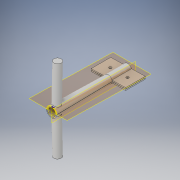
# Autodesk Inventor part: golfhandle
Saved by Autodesk Inventor 2018 (Build 220112000, 112)
## iProperties
Created: 2019-04-25
Part Number: golfhandle
Material: Generic
Document SubType Name: Modeling
Designer: F8PLTW
Density: 1 g/cm^3
Appearance: Default
Author: F8PLTW
Autodesk Inventor part; units mm, degrees
ref_plane "YZ Plane" through (0, 0, 0) normal (1, 0, 0) x (0, 1, 0)
ref_plane "XZ Plane" through (0, 0, 0) normal (0, 1, 0) x (-1, 0, 0)
ref_plane "XY Plane" through (0, 0, 0) normal (0, 0, 1) x (1, 0, 0)
sketch "Sketch1" plane through (0, 0, 0) normal (0, 0, 1) x (1, 0, 0)
  circle A0 centre (-3.872676, 4.498262) radius 10.795
  point P0 (0, 0)
  dimension "d0" = 21.59
  constraints: 1 centre point
  measures "d0" diameter of A0
extrude "Extrusion1" add sketch "Sketch1" along normal blind 2.54
ref_plane "Work Plane1" through (-3.872676, 4.498262, 156.718) normal (0, 0, 1) x (1, 0, 0)
sketch "Sketch2" plane through (-3.872676, 4.498262, 156.718) normal (0, 0, 1) x (1, 0, 0)
  circle A0 centre (0, 0) radius 13.716
  point P0 (3.872676, -4.498262)
  dimension "d4" = 27.432
  constraints: 1 centre point
  measures "d4" diameter of A0
loft "Loft1" add profiles "Sketch2" section 1 edges at (-14.667676, 4.498262, 2.54)
sketch "Sketch3" plane through (-3.872676, 4.498262, 0) normal (0, 0, -1) x (-1, 0, 0)
  circle A0 centre (0, 0) radius 10.795
  point P0 (-3.872676, -4.498262)
  dimension "d11" = 21.59
  constraints: 1 centre point
  measures "d11" diameter of A0
extrude "Extrusion2" add sketch "Sketch3" along normal blind 50.8
sketch "Sketch4" plane through (-3.872676, 4.498262, -50.8) normal (0, 0, -1) x (-1, 0, 0)
  point P0 (-3.872676, -4.498262)
sketch "Sketch5" plane through (-3.872676, 4.498262, -50.8) normal (0, 0, -1) x (-1, 0, 0)
  circle A0 centre (0, 0) radius 7.874
  point P0 (-3.872676, -4.498262)
  dimension "d12" = 15.748
  constraints: 1 centre point
  measures "d12" diameter of A0
extrude "Extrusion3" cut sketch "Sketch5" against normal blind 50.8
sketch "Sketch6" plane through (-3.872676, 4.498262, 0) normal (0, 0, -1) x (-1, 0, 0)
  circle A0 centre (0, 0) radius 7.62
  point P0 (-3.872676, -4.498262)
  constraints: 1 centre point
sketch "Sketch7" plane through (-3.872676, 4.498262, 156.718) normal (0, 0, 1) x (1, 0, 0)
  circle A0 centre (0, 0) radius 11.176
  point P0 (3.872676, -4.498262)
  dimension "d15" = 22.352
  constraints: 1 centre point
  measures "d15" diameter of A0
loft "Loft2" cut profiles "Sketch6", "Sketch7"
sketch "Sketch8" plane through (-3.872676, 4.498262, 0) normal (0, 0, -1) x (-1, 0, 0)
  circle A0 centre (0, 0) radius 7.874
  point P0 (-3.872676, -4.498262)
  constraints: 1 centre point
extrude "Extrusion4" cut sketch "Sketch8" against normal blind 2.54
sketch "Sketch9" plane through (-3.872676, 4.498262, 156.718) normal (0, 0, 1) x (1, 0, 0)
  line L0 (-5.096602, 0.25034) -> (248.903398, 0.25034)
  line L1 (248.903398, 0.25034) -> (248.903398, -0.25766)
  line L2 (248.903398, -0.25766) -> (-5.096602, -0.25766)
  line L3 (-5.096602, 0.25034) -> (-18.65647, 0.25034)
  line L4 (-5.096602, -0.25766) -> (-18.65647, -0.25766)
  line L5 (-18.65647, -0.25766) -> (-18.65647, 0.25034)
  point P0 (3.872676, -4.498262)
  dimension "d24" = 0.508
  dimension "d25" = 254
  constraints: 12 end point, 3 horizontal, 2 perpendicular, 1 parallel
  measures "d24" distance between parallel lines of L2 L0
  measures "d25" distance of L0.start L0.end
extrude "Extrusion5" cut sketch "Sketch9" against normal blind 228.6
ref_plane "Work Plane2" through (6.919421, 4.748602, 0) normal (0.9997311, 0.0231904, 0) x (-0.0231904, 0.9997311, 0)
sketch "Sketch10" plane through (6.919421, 4.748602, 0) normal (0.9997311, 0.0231904, 0) x (-0.0231904, 0.9997311, 0)
  line L0 (10.795, 2.54) -> (0, 2.54)
  line L1 (-0.075087, -50.8) -> (-7.874, -50.8)
  line L2 (3.133931, 2.54) -> (-0.075087, 2.54)
  line L3 (-0.075087, 2.54) -> (-0.075087, -50.8)
  line L4 (-0.075087, -50.8) -> (3.133931, -50.8)
  line L5 (3.133931, -50.8) -> (3.133931, 2.54)
  line L6 (-0.435537, 2.54) -> (-3.635937, 2.54)
  line L7 (-3.635937, 2.54) -> (-3.635937, -50.8)
  line L8 (-3.635937, -50.8) -> (-0.435537, -50.8)
  line L9 (-0.435537, -50.8) -> (-0.435537, 2.54)
  point P0 (-4.586861, 0)
  point P1 (0.500546, 2.54)
  point P2 (-0.440094, -50.8)
  dimension "d26" = 3.2004
  constraints: 16 end point, 4 parallel, 2 horizontal, 2 perpendicular, 2 point on line
  measures "d26" distance of L8.end L7.end
extrude "Extrusion6" add sketch "Sketch10" along normal mid plane 114.3
sketch "Sketch11" plane through (-50.287887, 6.556359, 2.54) normal (-0.0231904, 0.9997311, 0) x (0.9997311, 0.0231904, 0)
  circle A0 centre (24.391895, 27.825278) radius 3.429
  point P0 (50.122318, 2.54)
  dimension "d29" = 6.858
  constraints: 1 centre point
  measures "d29" diameter of A0
extrude "Extrusion7" cut sketch "Sketch11" against normal blind 50.8
sketch "Sketch12" plane through (6.381947, 7.870908, 2.54) normal (-0.0231904, 0.9997311, 0) x (0.9997311, 0.0231904, 0)
  line L0 (-18.20372, 0) -> (57.614922, 0)
  line L1 (-18.20372, 53.34) -> (57.614922, 53.34)
  line L2 (57.614922, 0) -> (37.396963, 0)
  line L3 (37.396963, 0) -> (37.396963, 53.34)
  line L4 (37.396963, 53.34) -> (57.614922, 53.34)
  line L5 (57.614922, 53.34) -> (57.614922, 0)
  point P0 (-6.56276, 2.54)
  constraints: 8 end point, 2 parallel, 1 horizontal, 1 perpendicular, 1 point on line
extrude "Extrusion8" cut sketch "Sketch12" against normal blind 50.8
sketch "Sketch13" plane through (6.381947, 7.870908, 2.54) normal (-0.0231904, 0.9997311, 0) x (0.9997311, 0.0231904, 0)
  circle A0 centre (15.500044, 27.091091) radius 3.429
  point P0 (-6.56276, 2.54)
  dimension "d34" = 6.858
  constraints: 1 centre point
  measures "d34" diameter of A0
extrude "Extrusion9" cut sketch "Sketch13" against normal blind 50.8
sketch "Sketch14" plane through (-3.872676, 4.498262, -50.8) normal (0, 0, -1) x (-1, 0, 0)
  circle A0 centre (0, 0) radius 7.874
  point P0 (-3.872676, -4.498262)
  constraints: 1 centre point
extrude "Extrusion10" cut sketch "Sketch14" against normal blind 63.5
sketch "Sketch15" plane through (-3.872676, 4.498262, -50.8) normal (0, 0, -1) x (-1, 0, 0)
  arc A0 (10.790094, -0.325401) -> (10.791925, -0.25766) centre (0, 0) ccw
  line L0 (-7.873266, 0.107526) -> (-47.715946, 1.031742)
  line L1 (10.791925, -0.25766) -> (-7.873266, 0.107526)
  arc A1 (-7.869783, -0.25766) -> (7.869783, -0.25766) centre (0, 0) ccw
  arc A2 (10.773209, -0.685557) -> (10.790094, -0.325401) centre (0, 0) ccw
  line L2 (-7.869783, -0.25766) -> (10.773209, -0.685557)
  line L3 (10.773209, -0.685557) -> (10.790094, -0.325401)
  line L4 (-7.873266, 0.107526) -> (-7.869783, -0.25766)
  point P0 (-3.872676, -4.498262)
  constraints: 8 end point
sketch "Sketch15 outline for Extrusion11" plane through (-3.872676, 4.498262, -50.8) normal (0, 0, -1) x (-1, 0, 0)
  arc A0 (10.790094, -0.325401) -> (10.791925, -0.25766) centre (0, 0) ccw
  line L0 (10.773209, -0.685557) -> (10.790094, -0.325401)
  line L1 (-7.869783, -0.25766) -> (10.773209, -0.685557)
  line L2 (-7.873266, 0.107526) -> (-7.869783, -0.25766)
  line L3 (10.791925, -0.25766) -> (-7.873266, 0.107526)
extrude "Extrusion11" cut sketch "Sketch15 outline for Extrusion11" against normal blind 304.8
sketch "Sketch16" plane through (-3.872676, 4.498262, 156.718) normal (0, 0, 1) x (1, 0, 0)
  arc A0 (13.713715, 0.25034) -> (-13.713715, 0.25034) centre (0, 0) ccw
  line L0 (0, 13.716) -> (8.803339, 13.716)
  point P0 (3.872676, -4.498262)
  constraints: 2 end point, 1 horizontal, 1 point on circle, 1 tangent
sketch "Sketch17" plane through (-3.872676, 4.498262, 156.718) normal (0, 0, 1) x (1, 0, 0)
  arc A0 (11.173196, 0.25034) -> (-11.173196, 0.25034) centre (0, 0) ccw
  line L0 (0, 11.176) -> (3.327889, 11.176)
  point P0 (3.872676, -4.498262)
  constraints: 2 end point, 1 horizontal, 1 point on circle, 1 tangent
ref_plane "Work Plane4" through (-3.872676, 15.674262, 156.718) normal (0, 0.9997427, -0.0226846) x (-1, 0, 0)
sketch "Sketch18" plane through (-3.872676, 15.674262, 156.718) normal (0, 0.9997427, -0.0226846) x (-1, 0, 0)
  ellipse E0 centre (0, -0.253523) end of major axis (13.716, -0.253523) minor radius 0.311142 (-13.71358, -0.259368) -> (13.71358, -0.259368) ccw
  line L0 (0, -0.253523) -> (0, -214.964518) construction
  circle A0 centre (0, -13.939044) radius 10.16
  point P0 (-3.872676, -157.033236)
  dimension "d41" = 20.32
  constraints: 2 end point, 1 centre point, 1 point on line, 1 vertical, 1 other
  measures "d41" diameter of A0
extrude "Extrusion12" add sketch "Sketch18" along normal blind 101.6
mirror "Mirror1" about plane through (-8.969278, 4.748602, 156.718) normal (0, -1, 0) of "Extrusion12"
sketch "Sketch19" plane through (-3.872676, 4.498262, 156.718) normal (0, 0, 1) x (1, 0, 0)
  circle A0 centre (0, 0) radius 11.176
  point P0 (3.872676, -4.498262)
  constraints: 1 centre point
extrude "Extrusion13" cut sketch "Sketch19" against normal blind 25.4
body "Solid1"
